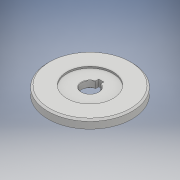
# Autodesk Inventor part: Hub Flange
Saved by Autodesk Inventor 2018 (Build 220112000, 112)
## iProperties
Created: 2018-03-27
Part Number: Hub Flange
Material: Generic
Document SubType Name: Modeling
Designer: P241310
Density: 1 g/cm^3
Appearance: Default
Author: P241310
Autodesk Inventor part; units mm, degrees
ref_plane "YZ Plane" through (0, 0, 0) normal (1, 0, 0) x (0, 1, 0)
ref_plane "XZ Plane" through (0, 0, 0) normal (0, 1, 0) x (-1, 0, 0)
ref_plane "XY Plane" through (0, 0, 0) normal (0, 0, 1) x (1, 0, 0)
sketch "Sketch1" plane through (0, 0, 0) normal (0, 0, 1) x (1, 0, 0)
  circle A0 centre (0, 0) radius 50
  dimension "d0" = 100
  constraints: 1 centre point, 1 coincident
  measures "d0" diameter of A0
extrude "Extrusion1" add sketch "Sketch1" along normal blind 10
sketch "Sketch2" plane through (0, 0, 10) normal (0, 0, 1) x (1, 0, 0)
  arc A0 (-3, 9.5394) -> (3, 9.5394) centre (0, 0) ccw
  line L0 (3, 9.5394) -> (3, 13.5)
  line L1 (3, 13.5) -> (-3, 13.5)
  line L2 (-3, 13.5) -> (-3, 9.5394)
  line L3 (-3, 6.5) -> (3, 13.5) construction
  line L4 (3, 6.5) -> (-3, 13.5) construction
  point P0 (0, 10)
  dimension "d3" = 20
  dimension "d4" = 6
  dimension "d5" = 3.5
  constraints: 10 end point, 2 midpoint, 2 point on circle, 1 centre point, 1 coincident, 1 parallel
  measures "d3" diameter of A0
  measures "d4" distance of L0.end L1.end
  measures "d5" vertical distance of point (0, 10) L0.end
extrude "Extrusion2" cut sketch "Sketch2" against normal blind 10
chamfer "Chamfer1" distance 2 angle 45 1 edges at (-50, 0, 10)
sketch "Sketch3" plane through (0, 0, 10) normal (0, 0, 1) x (1, 0, 0)
  circle A0 centre (0, 0) radius 27.5
  dimension "d11" = 55
  constraints: 1 centre point, 1 coincident
  measures "d11" diameter of A0
extrude "Extrusion3" cut sketch "Sketch3" against normal blind 2
chamfer "Chamfer2" distance 0.5 angle 45 2 edges at (0, -10, 0) (0, -10, 8)
body "Solid1"
